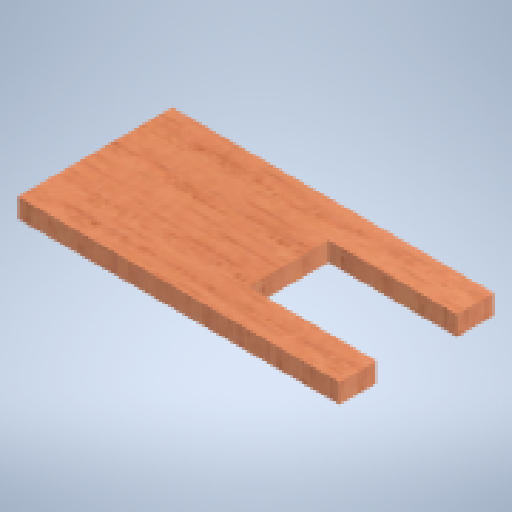
# Autodesk Inventor part: Mausefallle
Saved by Autodesk Inventor 2023 (Build 270158000, 158)
## iProperties
Created: 2023-02-17
Part Number: Mausefallle
Material: Wood (Oak)
Document SubType Name: Modeling
Designer: phill
Density: 0.76 g/cm^3
Appearance: White Oak - Natural Medium Gloss
Author: phill
Autodesk Inventor part; units mm, degrees
ref_plane "YZ Plane" through (0, 0, 0) normal (1, 0, 0) x (0, 1, 0)
ref_plane "XZ Plane" through (0, 0, 0) normal (0, 1, 0) x (-1, 0, 0)
ref_plane "XY Plane" through (0, 0, 0) normal (0, 0, 1) x (1, 0, 0)
sketch "Sketch1" plane through (0, 0, 0) normal (0, 1, 0) x (-1, 0, 0)
  line L0 (-50, 24) -> (50, 24)
  line L1 (50, 24) -> (50, -24)
  line L2 (50, -24) -> (-50, -24)
  line L3 (-50, -24) -> (-50, 24)
  point P0 (0, 0)
  point P1 (-50, 0)
  point P2 (0, 24)
  point P3 (-5, -14)
  dimension "d0" = 100
  dimension "d1" = 48
  dimension "d4" = 45
  dimension "d5" = 10
  constraints: 8 end point, 2 midpoint, 2 parallel, 1 horizontal, 1 horizontal alignment, 1 perpendicular, 1 vertical alignment
  measures "d0" distance of L0.start L0.end
  measures "d1" distance of L0.end L1.end
  measures "d4" distance from line of L3 point (-5, -14)
  measures "d5" distance from line of L2 point (-5, -14)
extrude "Extrusion1" add sketch "Sketch1" against normal blind 6
sketch "Sketch2" plane through (0, 0, 0) normal (0, 1, 0) x (1, 0, 0)
  line L0 (50, 24) -> (-50, 24) projected
  line L1 (-50, 24) -> (-50, -24) projected
  line L2 (-50, -24) -> (50, -24) projected
  line L3 (50, -24) -> (50, 24) projected
  line L4 (50, 24) -> (50, -24) projected
  line L5 (50, -12.5) -> (10, -12.5)
  line L6 (10, -12.5) -> (10, 12.5)
  line L7 (10, 12.5) -> (50, 12.5)
  line L8 (50, 12.5) -> (50, -12.5)
  point P0 (0, 0)
  point P1 (10, 0)
  dimension "d6" = 40
  dimension "d7" = 25
  constraints: 8 end point, 2 parallel, 1 horizontal, 1 horizontal alignment, 1 midpoint, 1 perpendicular, 1 point on line
  measures "d6" distance between parallel lines of L3 L6
  measures "d7" distance between parallel lines of L7 L5
extrude "Extrusion2" cut sketch "Sketch2" against normal blind 6 contours L3 L5 L6 L7
sketch "Sketch4" plane through (50, 0, -24) normal (0, 0, -1) x (-1, 0, 0)
  line L0 (0, 0) -> (0, -6) projected
  point P0 (50, 0)
  point P1 (10, -3)
  point P2 (0, -3)
  dimension "d12" = 10
  constraints: 1 horizontal alignment, 1 midpoint
  measures "d12" distance from line of L0 point (10, -3)
hole "Hole1" at (40, -3, -24) direction (0, 0, 1) diameter 3 end through all
body "Solid1"
